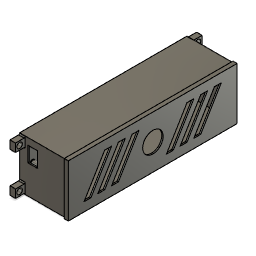
Коробка под электроннику v7 (Autodesk Fusion 360 design; units mm, degrees)
Autodesk Fusion 360 part; units mm, degrees
sketch "Sketch1" plane through (0, 0, 0) normal (1, 0, 0) x (0, 0, -1)
  line L0 (0, 0) -> (-120, 0)
  line L1 (-120, 0) -> (-120, 35)
  line L2 (-120, 35) -> (0, 35)
  line L3 (0, 35) -> (0, 0)
  line L4 (-120, 35) -> (-128, 35)
  line L5 (-128, 35) -> (-128, 29)
  line L6 (-128, 29) -> (-120, 29)
  line L7 (-120, 29) -> (-120, 35)
  line L8 (-120, 0) -> (-128, 0)
  line L9 (-128, 0) -> (-128, 6)
  line L10 (-128, 6) -> (-120, 6)
  line L11 (-120, 6) -> (-120, 0)
  line L12 (0, 35) -> (8, 35)
  line L13 (8, 35) -> (8, 29)
  line L14 (8, 29) -> (0, 29)
  line L15 (0, 29) -> (0, 35)
  line L16 (0, 0) -> (8, 0)
  line L17 (8, 0) -> (8, 6)
  line L18 (8, 6) -> (0, 6)
  line L19 (0, 6) -> (0, 0)
  circle A0 centre (5, 32) radius 2
  circle A1 centre (5, 3) radius 2
  circle A2 centre (-125, 3) radius 2
  circle A3 centre (-125, 32) radius 2
  dimension "d1" = 120
  dimension "d2" = 35
  dimension "d31" = 8
  dimension "d32" = 6
  dimension "d33" = 8
  dimension "d34" = 6
  dimension "d35" = 8
  dimension "d36" = 6
  dimension "d37" = 8
  dimension "d38" = 6
  dimension "d39" = 4
  dimension "d40" = 4
  dimension "d41" = 4
  dimension "d42" = 4
  constraint horizontal L0
  constraint vertical L1
  constraint horizontal L2
  constraint vertical L3
  constraint coincident L0.start L3.end
  constraint horizontal L4
  constraint vertical L5
  constraint horizontal L6
  constraint vertical L7
  constraint horizontal L8
  constraint vertical L9
  constraint horizontal L10
  constraint vertical L11
  constraint horizontal L12
  constraint vertical L13
  constraint horizontal L14
  constraint vertical L15
  constraint horizontal L16
  constraint vertical L17
  constraint horizontal L18
  constraint vertical L19
  measures "d1" distance of L0.start L0.end
  measures "d2" distance of L0.start L2.end
  measures "d31" distance of L1.end L4.end
  measures "d32" distance of L1.end L6.end
  measures "d33" distance of L0.end L8.end
  measures "d34" distance of L0.end L10.end
  measures "d35" distance of L2.end L12.end
  measures "d36" distance of L2.end L14.end
  measures "d37" distance of L0.start L16.end
  measures "d38" distance of L0.start L18.end
  measures "d39" diameter of A0
  measures "d40" diameter of A1
  measures "d41" diameter of A2
  measures "d42" diameter of A3
extrude "Extrude1" add sketch "Sketch1" along normal blind 5 contours L0 L1 L2 L3 L7 L11 L15 L19
sketch "Sketch2" plane through (5, 0, 0) normal (1, 0, 0) x (0, 0, -1)
  line L0 (0, 35) -> (-120, 35)
  line L1 (-120, 35) -> (-120, 0)
  line L2 (-120, 0) -> (0, 0)
  line L3 (0, 0) -> (0, 35)
  circle A0 centre (-62.2419, 32.2487) radius 1.5
  circle A1 centre (-7.2138, 32.2487) radius 1.5
  circle A2 centre (-7.2138, 4.2761) radius 1.5
  circle A3 centre (-62.2928, 4.2761) radius 1.5
  circle A4 centre (-116.5839, 32.3262) radius 1
  circle A5 centre (-75.9955, 32.3262) radius 1
  circle A6 centre (-75.9955, 17.7232) radius 1
  circle A7 centre (-116.621, 17.7232) radius 1
  circle A8 centre (-7.2138, 4.2761) radius 2.25
  circle A9 centre (-7.2138, 32.2487) radius 2.25
  circle A10 centre (-62.2928, 4.2761) radius 2.25
  circle A11 centre (-62.2419, 32.2487) radius 2.25
  circle A12 centre (-75.9955, 32.3262) radius 1.5
  circle A13 centre (-75.9955, 17.7232) radius 1.5
  circle A14 centre (-116.621, 17.7232) radius 1.5
  circle A15 centre (-116.5839, 32.3262) radius 1.5
  dimension "d5" = 3
  dimension "d6" = 3
  dimension "d7" = 3
  dimension "d8" = 3
  dimension "d9" = 2
  dimension "d10" = 2
  dimension "d11" = 2
  dimension "d12" = 2
  dimension "d13" = 4.5
  dimension "d14" = 4.5
  dimension "d15" = 4.5
  dimension "d16" = 4.5
  dimension "d17" = 3
  dimension "d18" = 3
  dimension "d19" = 3
  dimension "d20" = 3
  constraint concentric A2 A8
  constraint concentric A1 A9
  constraint concentric A3 A10
  constraint concentric A0 A11
  constraint concentric A5 A12
  constraint concentric A6 A13
  constraint concentric A7 A14
  constraint concentric A4 A15
  measures "d5" diameter of A0
  measures "d6" diameter of A1
  measures "d7" diameter of A2
  measures "d8" diameter of A3
  measures "d9" diameter of A4
  measures "d10" diameter of A5
  measures "d11" diameter of A6
  measures "d12" diameter of A7
  measures "d13" diameter of A8
  measures "d14" diameter of A9
  measures "d15" diameter of A10
  measures "d16" diameter of A11
  measures "d17" diameter of A12
  measures "d18" diameter of A13
  measures "d19" diameter of A14
  measures "d20" diameter of A15
extrude "Extrude2" cut sketch "Sketch2" against normal blind 30 contours A0 | A1 | A2 | A3 | A4 | A5 | A6 | A7
extrude "Extrude3" add sketch "Sketch2" along normal blind 2 contours A8 | A9 | A10 | A11 | A12 | A13 | A14 | A15
fillet "Fillet1" radius 0.3 8 edges at (5, 32.8686, 117.9824) (5, 18.2657, 118.0194) (5, 18.2657, 77.394) (5, 32.8686, 77.394) (5, 5.0897, 64.3906) (5, 5.0897, 9.3115) (5, 33.0624, 9.3115) (5, 33.0624, 64.3396)
sketch "Sketch3" plane through (5, 0, 0) normal (1, 0, 0) x (0, 0, -1)
  line L0 (1, -1) -> (-121, -1)
  line L1 (-121, -1) -> (-121, 36)
  line L2 (-121, 36) -> (1, 36)
  line L3 (1, 36) -> (1, -1)
  line L4 (-120, 35) -> (0, 35)
  line L5 (0, 35) -> (0, 0)
  line L6 (0, 0) -> (-120, 0)
  line L7 (-120, 0) -> (-120, 35)
  constraint horizontal L0
  constraint vertical L1
  constraint horizontal L2
  constraint vertical L3
  constraint horizontal L4
  constraint vertical L5
  constraint horizontal L6
  constraint vertical L7
  constraint coincident L5.end L6.start
extrude "Extrude4" add sketch "Sketch3" along normal blind 30 and the other way blind 5
extrude "Extrude6" add sketch "Sketch1" along normal blind 4 contours L3 L16 L17 L18 L19 | L1 L8 L9 L10 L11 | L3 L12 L13 L14 L15 | L1 L4 L5 L6 L7
fillet "Fillet2" radius 0.75 8 edges at (2, 29, -1) (2, 35, -1) (2, 6, -1) (2, 0, -1) (2, 0, 121) (2, 6, 121) (2, 29, 121) (2, 35, 121)
extrude "Extrude7" add 4 faces at (7, 32.6463, 115.2932) (7, 16.46, 117.0367) (7, 33.1357, 77.0506) (7, 17.6487, 74.6678) along direction (1, 0, 0) blind 4
sketch "Sketch4" plane through (0, 0, 121) normal (0, 0, 1) x (1, 0, 0)
  line L0 (0, 35.75) -> (4, 35.75)
  line L1 (4, 35.75) -> (4, 28.25)
  line L2 (4, 28.25) -> (0, 28.25)
  line L3 (0, 28.25) -> (0, 6.75)
  line L4 (0, 6.75) -> (4, 6.75)
  line L5 (4, 6.75) -> (4, -0.75)
  line L6 (4, -0.75) -> (0, -0.75)
  line L7 (0, -0.75) -> (0, -1)
  line L8 (0, -1) -> (35, -1)
  line L9 (35, -1) -> (35, 36)
  line L10 (35, 36) -> (0, 36)
  line L11 (0, 36) -> (0, 35.75)
  line L12 (6, 31.1165) -> (13, 31.1165)
  line L13 (13, 31.1165) -> (13, 20.0093)
  line L14 (13, 20.0093) -> (6, 20.0093)
  line L15 (6, 20.0093) -> (6, 31.1165)
  constraint horizontal L12
  constraint vertical L13
  constraint horizontal L14
  constraint vertical L15
extrude "Extrude8" cut sketch "Sketch4" against normal blind 1 contours L12 L13 L14 L15
sketch "Sketch5" plane through (0, 0, 121) normal (0, 0, 1) x (1, 0, 0)
sketch "Sketch6" plane through (0, 0, -1) normal (0, 0, -1) x (-1, 0, 0)
  line L0 (0, -0.75) -> (-4, -0.75)
  line L1 (-4, -0.75) -> (-4, 6.75)
  line L2 (-4, 6.75) -> (0, 6.75)
  line L3 (0, 6.75) -> (0, 28.25)
  line L4 (0, 28.25) -> (-4, 28.25)
  line L5 (-4, 28.25) -> (-4, 35.75)
  line L6 (-4, 35.75) -> (0, 35.75)
  line L7 (0, 35.75) -> (0, 36)
  line L8 (0, 36) -> (-35, 36)
  line L9 (-35, 36) -> (-35, -1)
  line L10 (-35, -1) -> (0, -1)
  line L11 (0, -1) -> (0, -0.75)
  line L12 (-15, 25) -> (-7, 25)
  line L13 (-7, 25) -> (-7, 10)
  line L14 (-7, 10) -> (-15, 10)
  line L15 (-15, 10) -> (-15, 25)
  constraint horizontal L12
  constraint vertical L13
  constraint horizontal L14
  constraint vertical L15
extrude "Extrude9" cut sketch "Sketch6" against normal blind 1 contours L12 L13 L14 L15
sketch "Sketch7" plane through (35, 0, 0) normal (1, 0, 0) x (0, 0, -1)
  line L0 (0, 0) -> (-120, 0)
  line L1 (-120, 0) -> (-120, 35)
  line L2 (-120, 35) -> (0, 35)
  line L3 (0, 35) -> (0, 0)
  line L4 (1, 36) -> (-121, 36)
  line L5 (-121, 36) -> (-121, -1)
  line L6 (-121, -1) -> (1, -1)
  line L7 (1, -1) -> (1, 36)
  line L8 (-121.5, 36.5) -> (1.5, 36.5)
  line L9 (1.5, 36.5) -> (1.5, -1.5)
  line L10 (1.5, -1.5) -> (-121.5, -1.5)
  line L11 (-121.5, -1.5) -> (-121.5, 36.5)
  constraint horizontal L8
  constraint vertical L9
  constraint horizontal L10
  constraint vertical L11
extrude "Extrude10" add sketch "Sketch7" along normal blind 1 contours L0 L1 L2 L3 | L4 L5 L6 L7 | L8 L9 L10 L11
extrude "Extrude11" add 1 faces at (35, 36.3333, 80.3333) along direction (-1, 0, 0) blind 2
sketch "Sketch8" plane through (36, 0, 0) normal (1, 0, 0) x (0, 0, -1)
  line L0 (-121.5, -1.5) -> (1.5, -1.5)
  line L1 (1.5, -1.5) -> (1.5, 36.5)
  line L2 (1.5, 36.5) -> (-121.5, 36.5)
  line L3 (-121.5, 36.5) -> (-121.5, -1.5)
  line L4 (-95, 30) -> (-110, 5)
  line L5 (-110, 5) -> (-105, 5)
  line L6 (-105, 5) -> (-90, 30)
  line L7 (-90, 30) -> (-95, 30)
  line L8 (-85, 30) -> (-80, 30)
  line L9 (-80, 30) -> (-95, 5)
  line L10 (-95, 5) -> (-100, 5)
  line L11 (-100, 5) -> (-85, 30)
  line L12 (-75, 30) -> (-70, 30)
  line L13 (-70, 30) -> (-85, 5)
  line L14 (-85, 5) -> (-90, 5)
  line L15 (-90, 5) -> (-75, 30)
  line L16 (-35, 30) -> (-30, 30)
  line L17 (-30, 30) -> (-45, 5)
  line L18 (-45, 5) -> (-50, 5)
  line L19 (-50, 5) -> (-35, 30)
  line L20 (-25, 30) -> (-20, 30)
  line L21 (-20, 30) -> (-35, 5)
  line L22 (-35, 5) -> (-40, 5)
  line L23 (-40, 5) -> (-25, 30)
  line L24 (-10, 30) -> (-25, 5)
  line L25 (-25, 5) -> (-30, 5)
  line L26 (-30, 5) -> (-15, 30)
  line L27 (-15, 30) -> (-10, 30)
  circle A0 centre (-59.8366, 17.5) radius 7.5
  dimension "d59" = 15
  constraint parallel L2 L5
  constraint parallel L4 L6
  constraint parallel L2 L7
  constraint parallel L7 L8
  constraint parallel L6 L9
  constraint parallel L8 L10
  constraint parallel L9 L11
  constraint parallel L8 L12
  constraint parallel L9 L13
  constraint parallel L12 L14
  constraint parallel L13 L15
  constraint parallel L12 L16
  constraint parallel L15 L17
  constraint parallel L12 L18
  constraint parallel L17 L19
  constraint parallel L16 L20
  constraint parallel L17 L21
  constraint horizontal L22
  constraint parallel L21 L23
  constraint parallel L21 L24
  constraint parallel L20 L25
  constraint parallel L24 L26
  constraint parallel L25 L27
  measures "d59" diameter of A0
extrude "Extrude12" cut sketch "Sketch8" against normal blind 5 contours L4 L5 L6 L7 | L8 L9 L10 L11 | L12 L13 L14 L15 | L16 L17 L18 L19 | L20 L21 L22 L23 | L24 L25 L26 L27 | A0
extrude "Extrude5" [suppressed]
